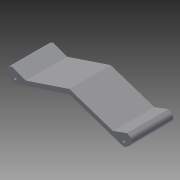
# Autodesk Inventor part: Front Support
Saved by Autodesk Inventor 2015 (Build 190159000, 159)
## iProperties
Created: 2016-08-02
Part Number: Front Support
Material: Generic
Document SubType Name: Modeling
Designer: James Yelland
Density: 1 g/cm^3
Appearance: Default
Author: James Yelland
Autodesk Inventor part; units mm, degrees
ref_plane "YZ Plane" through (0, 0, 0) normal (1, 0, 0) x (0, 1, 0)
ref_plane "XZ Plane" through (0, 0, 0) normal (0, 1, 0) x (-1, 0, 0)
ref_plane "XY Plane" through (0, 0, 0) normal (0, 0, 1) x (1, 0, 0)
sketch "Sketch1" plane through (0, 0, 0) normal (0, 1, 0) x (-1, 0, 0)
  line L0 (62.8442, -65.1506) -> (65.5625, -66.72)
  line L1 (-62.8442, -65.1506) -> (-65.5625, -66.72)
  arc A0 (66.3816, -74.7896) -> (65.5625, -66.72) centre (63.0625, -71.0502) ccw
  arc A1 (-65.5625, -66.72) -> (-66.3816, -74.7896) centre (-63.0625, -71.0502) ccw
  line L2 (0, -60) -> (-57.4738, -79.1579)
  line L3 (0, -60) -> (57.4738, -79.1579)
  arc A2 (62.1631, -78.3311) -> (66.3816, -74.7896) centre (0, 0) ccw
  arc A3 (-66.3816, -74.7896) -> (-62.1631, -78.3311) centre (0, 0) ccw
  arc A4 (57.4738, -79.1579) -> (62.1631, -78.3311) centre (59.0549, -74.4145) ccw
  arc A5 (-62.1631, -78.3311) -> (-57.4738, -79.1579) centre (-59.0549, -74.4145) ccw
  circle A6 centre (59.0549, -74.4145) radius 1.6
  circle A7 centre (-59.0549, -74.4145) radius 1.6
  line L4 (0, -55) -> (-47.4342, -70.8114)
  line L5 (-62.8442, -65.1506) -> (-47.4342, -70.8114)
  line L6 (0, -55) -> (47.4342, -70.8114)
  line L7 (47.4342, -70.8114) -> (62.8442, -65.1506)
  point P0 (0, 0)
  point P1 (71.3525, -70.0629)
  point P2 (86.1122, -20.8494)
  point P3 (-71.3525, -70.0629)
  point P4 (-86.1122, -20.8494)
  point P5 (60, -80)
  point P6 (-60, -80)
  dimension "d3" = 5
  dimension "d4" = 3.2
  dimension "d5" = 3.2
  dimension "d7" = 50
  constraints: 16 end point, 14 point on circle, 8 centre point, 6 tangent, 4 point on line, 3 coincident, 1 equal radius, 1 parallel
  measures "d3" radius of A4
  measures "d4" diameter of A6
  measures "d5" diameter of A7
  measures "d7" distance of L4.start L4.end
extrude "Extrusion1" add sketch "Sketch1" along normal blind 45
body "Solid1"
